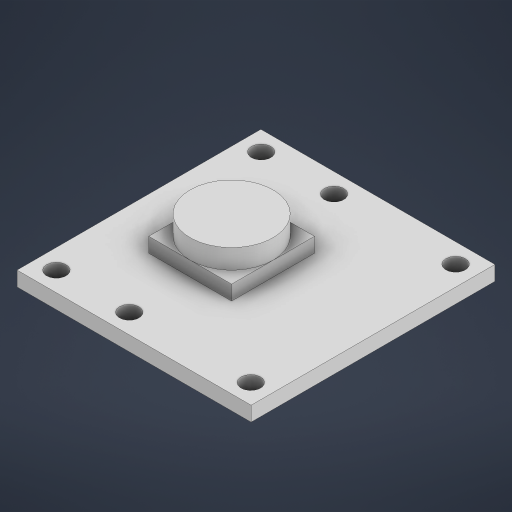
# Autodesk Inventor part: pasapery pi camera
Saved by Autodesk Inventor 2024 (Build 280153000, 153)
## iProperties
Created: 2023-06-15
Part Number: pasapery pi camera
Material: 일반
Document SubType Name: Modeling
Designer: 6gioc
Density: 1 g/cm^3
Appearance: 기본값
Author: 6gioc
Autodesk Inventor part; units mm, degrees
ref_plane "YZ Plane" through (0, 0, 0) normal (1, 0, 0) x (0, 1, 0)
ref_plane "XZ Plane" through (0, 0, 0) normal (0, 1, 0) x (-1, 0, 0)
ref_plane "XY Plane" through (0, 0, 0) normal (0, 0, 1) x (1, 0, 0)
sketch "스케치1" plane through (0, 0, 0) normal (0, 1, 0) x (-1, 0, 0)
  line L0 (0, 0) -> (24, 0)
  line L1 (24, 0) -> (24, -25)
  line L2 (24, -25) -> (0, -25)
  line L3 (0, -25) -> (0, 0)
  circle A0 centre (21.97, -2) radius 1
  circle A1 centre (2.03, -2) radius 1
  circle A2 centre (14.5, -2) radius 1
  circle A3 centre (21.97, -23) radius 1
  circle A4 centre (14.5, -23) radius 1
  circle A5 centre (2.03, -23) radius 1
  line L4 (18.75, -8.25) -> (10.25, -8.25)
  line L5 (10.25, -8.25) -> (10.25, -16.75)
  line L6 (10.25, -16.75) -> (18.75, -16.75)
  line L7 (18.75, -16.75) -> (18.75, -8.25)
  circle A6 centre (14.5, -12.5) radius 4.25
  point P0 (0, -12.5)
  point P1 (14.5, -8.25)
  point P2 (18.75, -12.5)
  point P3 (14.5, -16.75)
  point P4 (10.25, -12.5)
  dimension "d0" = 24
  dimension "d1" = 25
  dimension "d2" = 2
  dimension "d3" = 2
  dimension "d4" = 2
  dimension "d5" = 2
  dimension "d7" = 2
  dimension "d8" = 2
  dimension "d9" = 2
  dimension "d10" = 2
  dimension "d11" = 2.03
  dimension "d12" = 2.03
  dimension "d13" = 21
  dimension "d14" = 21
  dimension "d15" = 21
  dimension "d16" = 14.5
  dimension "d17" = 14.5
  dimension "d18" = 2.03
  dimension "d19" = 2.03
  dimension "d23" = 8.5
  dimension "d24" = 8.5
  dimension "d25" = 14.5
  dimension "d26" = 12.5
  constraints: 16 end point, 7 centre point, 4 parallel, 3 tangent, 2 horizontal, 2 perpendicular, 1 midpoint
  measures "d0" distance of L1.end L2.end
  measures "d1" distance of L0.end L1.end
  measures "d2" diameter of A0
  measures "d3" diameter of A1
  measures "d4" diameter of A2
  measures "d5" diameter of A3
  measures "d7" diameter of A5
  measures "d8" distance from line of L0 A1.centre
  measures "d9" distance from line of L0 A2.centre
  measures "d10" distance from line of L0 A0.centre
  measures "d11" distance from line of L3 A1.centre
  measures "d12" distance from line of L3 A5.centre
  measures "d13" distance of A5.centre A1.centre
  measures "d14" distance of A4.centre A2.centre
  measures "d15" distance of A0.centre A3.centre
  measures "d16" distance from line of L3 A4.centre
  measures "d17" distance from line of L3 A2.centre
  measures "d18" distance from line of L1 A0.centre
  measures "d19" distance from line of L1 A3.centre
  measures "d23" distance of L6.end L5.end
  measures "d24" distance of L5.end L4.end
  measures "d25" distance from line of L3 A6.centre
  measures "d26" distance from line of L0 A6.centre
extrude "돌출1" add sketch "스케치1" along normal blind 1.5
extrude "돌출2" add sketch "스케치1" along normal blind 3 contours L7 A6 L4 | A6 L5 L4 | L7 L6 A6 | A6 L6 L5
extrude "돌출3" add sketch "스케치1" along normal blind 5 contours A6
